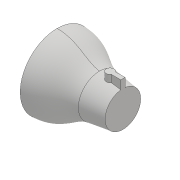
# Autodesk Inventor part: Lamp_Shade
Saved by Autodesk Inventor 2018 (Build 220112000, 112)
## iProperties
Created: 2019-09-21
Part Number: Lamp_Shade
Material: Generic
Document SubType Name: Modeling
Designer: Clevo
Density: 1 g/cm^3
Appearance: Default
Author: Clevo
Autodesk Inventor part; units mm, degrees
ref_plane "YZ Plane" through (0, 0, 0) normal (1, 0, 0) x (0, 1, 0)
ref_plane "XZ Plane" through (0, 0, 0) normal (0, 1, 0) x (-1, 0, 0)
sketch "Sketch1" plane through (0, 0, 0) normal (0, 1, 0) x (-1, 0, 0)
  line L0 (62.5, 0) -> (-62.5, 0)
  line L1 (-62.5, 0) -> (-17.9379, 0)
  line L2 (-17.9379, 0) -> (-17.9379, 40)
  line L3 (-62.5, 33.7372) -> (-62.5, 0)
  line L4 (-17.9379, 40) -> (10, 45) construction
  line L5 (10, 45) -> (22, 70) construction
  line L6 (22, 70) -> (62.5, 70) construction
  spline S0 degree 3 poles (-17.9379, 40) (10, 45) (22, 70) (62.5, 70) knots 1 1 1 1 2 2 2 2
  line L7 (62.5, 70) -> (62.5, 0)
  line L8 (-62.5, 33.7372) -> (-17.9379, 40)
  point P0 (0, 0)
  point P1 (0, 0)
  dimension "d0" = 125
  dimension "d1" = 40
  dimension "d2" = 45
  dimension "d3" = 45
  dimension "d4" = 10
  dimension "d5" = 70
  dimension "d6" = 22
  dimension "d7" = 70
  dimension "d9" = 98
  constraints: 12 end point, 2 horizontal, 1 coincident, 1 midpoint, 1 parallel, 1 perpendicular, 1 vertical, 1 vertical alignment, 3 other
  measures "d0" distance of L0.start L0.end
  measures "d1" distance of L1.end L2.end
  measures "d2" distance of L2.end L3.start
  measures "d3" distance from line of L0 L4.end
  measures "d4" horizontal distance of L4.end point (0, 0)
  measures "d5" vertical distance of point (0, 0) L5.end
  measures "d6" horizontal distance of point (0, 0) L5.end
  measures "d7" distance from line of L0 L6.end
  measures "d9" angle of L8 L3
revolve "Revolution1" add sketch "Sketch1" angle 360 about axis through (-62.5, 0, 0) along (1, 0, 0)
ref_plane "Work Plane1" through (0, 0, 50) normal (0, 0, 1) x (1, 0, 0)
sketch "Sketch2" plane through (0, 0, 50) normal (0, 0, 1) x (1, 0, 0)
  circle A0 centre (38, 0) radius 7.5
  point P0 (0, 0)
  dimension "d15" = 15
  dimension "d16" = 38
  constraints: 1 centre point, 1 horizontal alignment
  measures "d15" diameter of A0
  measures "d16" distance of A0.centre point (0, 0)
extrude "Extrusion1" add sketch "Sketch2" against normal up to surface round surface about axis through (40.219, 0, 0) along (-1, 0, 0) radius 36.8686 half angle 8 far side no
sketch "Sketch6" plane through (38, 0, 50) normal (0, 0, 1) x (1, 0, 0)
  circle A0 centre (0, 0) radius 7.5 projected
  line L0 (24.5, 33.7372) -> (24.5, -33.7372) projected
  line L1 (24.5, -4) -> (4.5, -4)
  line L2 (4.5, -4) -> (4.5, 4)
  line L3 (4.5, 4) -> (24.5, 4)
  line L4 (24.5, 4) -> (24.5, -4)
  point P0 (-38, 0)
  dimension "d39" = 20
  constraints: 8 end point, 2 parallel, 1 horizontal, 1 perpendicular, 1 point on line
  measures "d39" distance of L1.start L1.end
extrude "Extrusion4" add sketch "Sketch6" against normal up to surface contours A0 L1 L2 L3 | A0 L3 L0 L1 round surface about axis through (40.219, 0, 0) along (-1, 0, 0) radius 36.8686 half angle 8 far side no picked at (5.5, 0)
body "Solid1"
